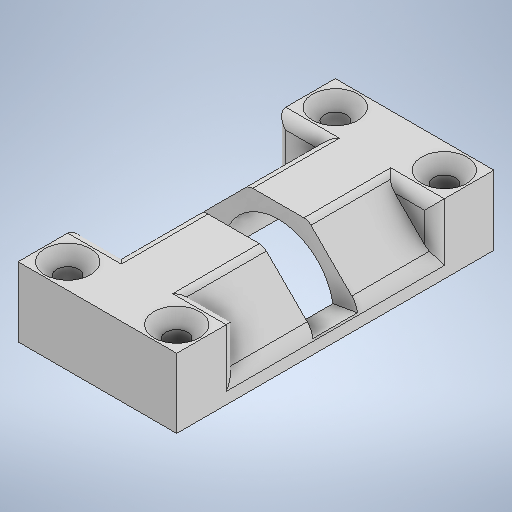
# Autodesk Inventor part: SwitchLeverUnit_UpperCase
Saved by Autodesk Inventor 2025.1 (Build 291241000, 241)
## iProperties
Created: 2025-03-09
Part Number: SwitchLeverUnit_UpperCase
Material: 一般
Document SubType Name: Modeling
Designer: kumagai
Density: 1 g/cm^3
Appearance: 既定
Author: kumagai
Autodesk Inventor part; units mm, degrees
ref_plane "YZ Plane" through (0, 0, 0) normal (1, 0, 0) x (0, 1, 0)
ref_plane "XZ Plane" through (0, 0, 0) normal (0, 1, 0) x (-1, 0, 0)
ref_plane "XY Plane" through (0, 0, 0) normal (0, 0, 1) x (1, 0, 0)
derived "SwitchLeverUnit_LowerCase.ipt"
sketch "DrumSketch" plane through (0, 0, 0) normal (0, 0, 1) x (1, 0, 0)
  line L0 (0, 8.12) -> (0, -9.52)
  line L1 (-7.84, 0) -> (7.84, 0)
  circle A0 centre (0, 0) radius 4.2
  line L2 (-2.7, -3) -> (2.7, -3)
  line L3 (2.7, 0) -> (2.7, -7)
  line L4 (2.7, -7) -> (-2.7, -7)
  line L5 (-2.7, -7) -> (-2.7, 0)
  circle A1 centre (0, 0) radius 5.6
sketch "BodySketch" plane through (0, 0, 0) normal (0, 1, 0) x (-1, 0, 0)
  line L0 (8, 16) -> (-8, 16)
  line L1 (-8, 16) -> (-8, -16)
  line L2 (-8, -16) -> (8, -16)
  line L3 (8, -16) -> (8, 16)
  line L4 (0, -38.6) -> (0, 25.1)
  line L5 (-11.2, 0) -> (11.2, 0)
  circle A0 centre (5.5, 13.5) radius 1.1
  circle A1 centre (5.5, 13.5) radius 1.65
  circle A2 centre (5.5, -13.5) radius 1.65
  circle A3 centre (5.5, -13.5) radius 1.1
  circle A4 centre (-5.5, 13.5) radius 1.65
  circle A5 centre (-5.5, 13.5) radius 1.1
  circle A6 centre (-5.5, -13.5) radius 1.1
  circle A7 centre (-5.5, -13.5) radius 1.65
  line L6 (7, -16) -> (7, -18)
  line L7 (7, -18) -> (6, -18)
  line L8 (6, -18) -> (8, -29.5)
  line L9 (8, -29.5) -> (-8, -29.5)
  line L10 (-8, -29.5) -> (-6, -18)
  line L11 (-6, -18) -> (-7, -18)
  line L12 (-7, -18) -> (-7, -16)
  line L13 (3.7, -29.5) -> (3.7, -16)
  line L14 (-3.7, -29.5) -> (-3.7, -16)
  line L15 (2.4888, -22.75) -> (1.2404, -22.75)
  circle A8 centre (5.5, 13.5) radius 1.75
  circle A9 centre (5.5, -13.5) radius 1.75
  circle A10 centre (-5.5, 13.5) radius 1.75
  circle A11 centre (-5.5, -13.5) radius 1.75
  point P0 (0, 0)
extrude "MainBody" add sketch "BodySketch" along normal blind 7 contours L3 L5 L4 L0 | L4 L5 L1 L0 | L3 L2 L4 L5 | L4 L2 L1 L5 | A1 | A2 | A4 | A7 | A8 | A9 | A10 | A11
extrude "RollerChannel" cut sketch "DrumSketch" along normal mid plane 22 contours A1 L1 A0 L0 | L0 A0 L1 A1 | A0 L1 L0 | L0 L1 A0 | A1 L3 A0 L1 | L1 A0 L5 A1 | L1 L3 L2 L0 | L0 L2 L5 L1 | A0 L3 L1 | L1 L5 A0 | A1 L0 A0 L3 | L5 A0 L0 A1 | L2 L3 A0 L0 | L0 A0 L5 L2
extrude "RollerBearing" cut sketch "DrumSketch" along normal mid plane 24.4 contours A0 L1 L0 | L0 L1 A0 | L1 L3 L2 L0 | L0 L2 L5 L1 | A0 L3 L1 | L1 L5 A0 | L2 L3 A0 L0 | L0 A0 L5 L2
chamfer "HoleChamfer" distance 1.2 angle 45 4 edges at (-4.4, 7, -13.5) (6.6, 7, -13.5) (-4.4, 7, 13.5) (6.6, 7, 13.5)
sketch "TopShape" plane through (0, 0, 0) normal (0, 0, 1) x (1, 0, 0)
  line L0 (-5.6, 0) -> (-8, 0) projected
  line L1 (-8, 0) -> (-8, 7) projected
  line L2 (-8, 7) -> (8, 7) projected
  line L3 (8, 7) -> (8, 0) projected
  line L4 (8, 0) -> (5.6, 0) projected
  arc A0 (5.6, 0) -> (-5.6, 0) centre (0, 0) ccw projected
  line L5 (-8, 2) -> (-3, 7)
  line L6 (3, 7) -> (8, 2)
  line L7 (0, 0) -> (-10.8333, 1.9102)
  line L8 (0, 0) -> (10.8333, 1.9102)
  arc A1 (10.8333, 1.9102) -> (-10.8333, 1.9102) centre (0, 0) ccw
  line L9 (0, 13.2005) -> (0, -2.2001) projected
  line L10 (-15.1666, 0) -> (15.1666, 0) projected
  dimension "d39" = 5
  dimension "d40" = 5
  dimension "d41" = 5
  dimension "d42" = 5
  dimension "d45" = 11.0004
  dimension "d46" = 10
  constraints: 8 end point, 4 point on line, 2 point on circle, 1 centre point, 1 coincident, 1 symmetric about line
  measures "d39" distance of L1.end L5.start
  measures "d40" distance from line of L5.end L1
  measures "d41" distance from line of L6.start L3
  measures "d42" distance from line of L6.end L2
  measures "d45" radius of A1
  measures "d46" angle of L10 L7
extrude "TopCut" cut sketch "TopShape" along normal mid plane 20 contours L1 L2 L5 | L2 L3 L6
extrude "LeverHole" cut sketch "TopShape" along normal mid plane 4.5 contours L7 L1 L5 L2 L9 A0 | A0 L9 L7 | L9 A0 L8 | L7 A1 L9 L2 L1 | L9 L2 L6 L3 L8 A0 | L1 L2 L5 | L9 A1 L8 L3 L2 | L2 L3 L6
fillet "Fillet1" radius 2 4 edges at (-8, 2, 6.125) (-8, 2, -6.125) (8, 2, 6.125) (8, 2, -6.125)
fillet "Fillet2" radius 1 13 edges at (5.5, 7, -10) (8, 4.0858, -10) (3, 7, -6.125) (3, 7, 6.125) (5.5, 7, 10) (8, 4.0858, 10) (-8, 1.5858, 10) (-8, 4.5, 10) (-5.5, 7, 10) (-3, 7, 6.125) (-3, 7, -6.125) (-5.5, 7, -10) (-8, 4.0858, -10)
equation "\"d40\" = d39"
equation "\"d41\" = d39"
equation "\"d42\" = d39"
